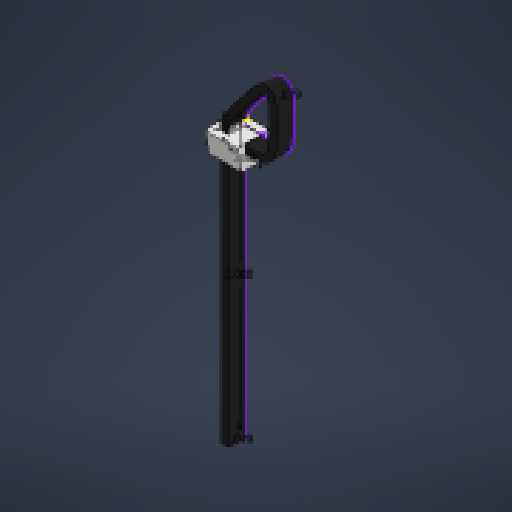
# Autodesk Inventor part: Cata zip tie
Saved by Autodesk Inventor 2023.2 (Build 272271030, 271C)
## iProperties
Created: 2023-05-29
Part Number: Cata zip tie
Material: Generic
Document SubType Name: Modeling
Designer: Main Account
Density: 1 g/cm^3
Appearance: Default
Author: Main Account
Autodesk Inventor part; units mm, degrees
ref_plane "YZ Plane" through (0, 0, 0) normal (1, 0, 0) x (0, 1, 0)
ref_plane "XZ Plane" through (0, 0, 0) normal (0, 1, 0) x (-1, 0, 0)
ref_plane "XY Plane" through (0, 0, 0) normal (0, 0, 1) x (1, 0, 0)
sketch "Sketch1" plane through (0, 0, 0) normal (0, 0, 1) x (1, 0, 0)
  line L0 (0, 0) -> (-3.6068, 0) construction
  line L1 (0, 0) -> (0, 1.5875)
  line L2 (-3.6068, 1.5875) -> (0, 1.5875) construction
  line L3 (-3.6068, 0) -> (-3.6068, 1.5875) construction
  line L4 (10.8966, 3.321) -> (10.8966, 13.3477) construction
  line L5 (10.8966, 14.2875) -> (10.8966, 13.2715) construction
  line L6 (9.3091, 14.2875) -> (10.8966, 14.2875) construction
  line L7 (10.8966, 3.3972) -> (10.8966, 2.3813) construction
  spline S0 degree 3 poles (10.8966, 2.3813) (10.8966, 1.718) (10.6045, 1.06) (10.1126, 0.6151) knots 0 0 0 0 1 1 1 1 construction
  spline S1 degree 3 poles (10.1126, 0.6151) (9.6798, 0.2237) (9.0989, 0) (8.5153, 0) knots 0 0 0 0 1 1 1 1 construction
  line L8 (-4.445, 0) -> (-4.445, -6.35)
  line L9 (-4.445, -6.35) -> (4.445, -6.35)
  line L10 (4.445, -6.35) -> (4.445, 0)
  spline S2 degree 4 poles (0, 1.5875) (0.0398, 3.838) (8.3304, 12.4869) (11.798, 20.7343) (11.181, 1.9788) (11.0427, -0.2379) (6.8946, -0.4139) (4.445, -0.2668) knots 0 0 0 0 0 0.396484 0.590569 0.753234 1 1 1 1 1
  line L11 (11.3428, 2.8356) -> (10.0194, -0.0386) construction
  arc A0 (9.9788, 0.4386) -> (10.9538, 2.5562) centre (7.964, 2.6496) ccw construction
  line L12 (-0.0202, 0.4489) -> (0.0202, 2.7261) construction
  arc A1 (0.2539, 2.3166) -> (0.228, 0.8499) centre (1.2364, 1.5656) ccw construction
  line L13 (0, 1.5875) -> (0, -74.6125)
  line L14 (0, -74.6125) -> (-2, -74.6125)
  line L15 (-2, -74.6125) -> (-2, 1.5875)
  line L16 (-1.9997, 1.6229) -> (-2, 1.5875)
  line L17 (7.7554, -0.4656) -> (1.1346, -0.0679) construction
  arc A2 (1.8128, 0.0031) -> (7.0906, -0.314) centre (6.3271, 31.0611) ccw construction
  line L18 (4.445, -2.2702) -> (1.1345, -2.0915)
  line L19 (4.445, -0.2668) -> (1.1345, -0.0882)
  line L20 (1.1345, -2.0915) -> (1.1345, -0.0882)
  line L21 (4.445, 0) -> (-4.445, 0)
  spline S3 degree 5 poles (-1.9997, 1.6229) (-1.9907, 2.1668) (-1.8639, 2.7081) (-1.6627, 3.2153) (-1.1799, 4.2153) (-0.5925, 5.1574) (-0.2813, 5.629) (0.3951, 6.6071) (1.1009, 7.564) (1.4765, 8.0623) (2.2352, 9.0534) (3.0062, 10.0352) (3.3939, 10.5243) (4.1368, 11.4534) (4.8885, 12.375) (5.248, 12.8113) (5.9112, 13.6043) (6.5923, 14.3831) (6.9065, 14.7305) (7.5274, 15.3927) (8.2052, 15.9938) (8.5504, 16.2662) (9.5346, 16.8442) (10.7011, 16.9465) (11.4362, 16.7212) (12.3745, 15.9613) (12.854, 14.8838) (12.9769, 14.4266) (13.1691, 13.4629) (13.2552, 12.4819) (13.288, 11.9711) (13.3342, 10.8672) (13.3468, 9.7633) (13.3468, 9.1713) (13.3384, 8.0057) (13.3143, 6.8401) (13.2992, 6.2663) (13.2636, 5.2008) (13.2042, 4.1362) (13.1694, 3.6455) (13.0826, 2.7071) (12.9164, 1.7798) (12.8117, 1.3413) (12.5093, 0.4586) (12.0101, -0.3303) (11.6939, -0.6986) (10.9887, -1.3082) (10.1543, -1.722) (9.732, -1.8759) (8.8714, -2.111) (7.9873, -2.2328) (7.5452, -2.273) (6.6596, -2.3224) (5.7727, -2.3222) (5.3298, -2.3127) (4.8872, -2.2951) (4.445, -2.2702) knots 0 0 0 0 0 0 0.057735 0.057735 0.057735 0.117738 0.117738 0.117738 0.183995 0.183995 0.183995 0.250287 0.250287 0.250287 0.310299 0.310299 0.310299 0.3601 0.3601 0.3601 0.406513 0.406513 0.406513 0.479615 0.479615 0.479615 0.529521 0.529521 0.529521 0.583941 0.583941 0.583941 0.64678 0.64678 0.64678 0.707734 0.707734 0.707734 0.759988 0.759988 0.759988 0.807705 0.807705 0.807705 0.858414 0.858414 0.858414 0.905852 0.905852 0.905852 0.952969 0.952969 0.952969 1 1 1 1 1 1
  point P0 (10.6811, 1.3985)
extrude "head part" add sketch "Sketch1" along normal blind 6.7564 and the other way blind 2.1336 contours L21 L10 L19 L20 L18 L9 L13 | L13 L9 L15 L21 | L15 L9 L8 L21 | L10 L18 L20 L19
sketch "Sketch2" plane through (4.445, -6.35, 6.7564) normal (1, 0, 0) x (0, 0, -1)
  line L0 (0, 0) -> (0, 6.35) projected
  line L1 (8.89, 0) -> (0, 0) projected
  line L2 (8.89, 6.35) -> (8.89, 0) projected
  line L3 (0, 6.35) -> (1.27, 0)
  line L4 (8.89, 6.35) -> (7.62, 0)
  dimension "d27" = 1.27
  dimension "d28" = 1.27
  constraints: 4 end point, 2 point on line
  measures "d27" distance of L1.start L4.end
  measures "d28" distance of L0.start L3.end
extrude "side cuts" cut sketch "Sketch2" against normal blind 8.89
sketch "Sketch4" plane through (0, 0, 0) normal (0, 0, 1) x (1, 0, 0)
  line L0 (4.445, -6.35) -> (4.445, 0) projected
  line L1 (-4.445, -6.35) -> (4.445, -6.35) projected
  line L2 (-4.445, 0) -> (-4.445, -6.35) projected
  line L3 (-4.445, -6.35) -> (-4.445, 0) projected
  line L4 (-4.445, 0) -> (-3.175, -6.35)
  line L5 (4.445, -6.35) -> (-4.445, -6.35) projected
  line L6 (3.175, -6.35) -> (4.445, 0)
  dimension "d29" = 1.27
  dimension "d30" = 1.27
  constraints: 4 end point, 2 point on line
  measures "d29" distance of L0.start L6.start
  measures "d30" distance of L1.start L4.end
extrude "top cuts" cut sketch "Sketch4" along normal through all both and the other way through all
extrude "tie part" add sketch "Sketch1" along normal blind 4.6228 contours L21 L15 L16 S3 L10 S2 L1 | L13 L9 L15 L21 | L13 L14 L15 L9 | L10 L18 L20 L19
body "Solid1"
